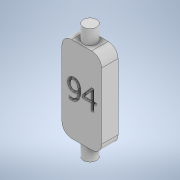
# Autodesk Inventor part: 16-2
Saved by Autodesk Inventor 2022 (Build 260153000, 153)
## iProperties
Created: 2021-09-25
Part Number: 16-2
Material: 일반
Document SubType Name: Modeling
Designer: 서울공업고등학교
Density: 1 g/cm^3
Appearance: 기본값
Author: 서울공업고등학교
Autodesk Inventor part; units mm, degrees
ref_plane "YZ Plane" through (0, 0, 0) normal (1, 0, 0) x (0, 1, 0)
ref_plane "XZ Plane" through (0, 0, 0) normal (0, 1, 0) x (-1, 0, 0)
ref_plane "XY Plane" through (0, 0, 0) normal (0, 0, 1) x (1, 0, 0)
sketch "스케치1" plane through (0, 0, 0) normal (0, 0, 1) x (1, 0, 0)
  line L0 (-6, 13) -> (6, 13)
  line L1 (6, 13) -> (6, -13)
  line L2 (6, -13) -> (-6, -13)
  line L3 (-6, -13) -> (-6, 13)
  line L4 (-6, 13) -> (6, -13) construction
  line L5 (6, 13) -> (-6, -13) construction
  point P0 (0, 0)
  dimension "d0" = 12
  dimension "d1" = 26
  constraints: 12 end point, 2 midpoint, 2 parallel, 1 horizontal, 1 perpendicular
  measures "d0" distance of L1.end L2.end
  measures "d1" distance of L0.end L1.end
extrude "돌출1" add sketch "스케치1" along normal mid plane 5
fillet "모깎기1" radius 3 4 edges at (6, 13, 0) (-6, 13, 0) (6, -13, 0) (-6, -13, 0)
sketch "스케치2" plane through (-3, 13, 2.5) normal (0, 1, 0) x (1, 0, 0)
  circle A0 centre (3, 2.5) radius 2
  dimension "d5" = 4
  constraints: 1 centre point, 1 coincident
  measures "d5" diameter of A0
extrude "돌출2" add sketch "스케치2" along normal blind 4.5 and the other way blind 30.5
sketch "스케치3" plane through (0, 0, 2.5) normal (0, 0, 1) x (1, 0, 0)
  line L0 (-4.5251, 3.4564) -> (4.6298, 3.4564) construction
  line L1 (4.6298, 3.4564) -> (4.6298, -2.8858) construction
  line L2 (4.6298, -2.8858) -> (-4.5251, -2.8858) construction
  line L3 (-4.5251, -2.8858) -> (-4.5251, 3.4564) construction
  spline S0 degree 2 poles (-4.2483, 1.3506) (-4.2483, 1.8202) (-3.9418, 2.6012) (-3.6749, 2.883) knots 0 0 0 1 2 2 2
  spline S1 degree 2 poles (-3.6749, 2.883) (-3.4228, 3.1549) (-2.6863, 3.4564) (-2.3106, 3.4564) knots 0 0 0 1 2 2 2
  spline S2 degree 2 poles (-2.3106, 3.4564) (-1.8904, 3.4564) (-1.2082, 3.1746) (-0.9561, 2.9077) knots 0 0 0 1 2 2 2
  spline S3 degree 2 poles (-0.9561, 2.9077) (-0.6397, 2.5715) (-0.2937, 1.484) (-0.2937, 0.6486) knots 0 0 0 1 2 2 2
  spline S4 degree 2 poles (-0.2937, 0.6486) (-0.2937, -0.1077) (-0.6348, -1.4622) (-0.966, -1.912) knots 0 0 0 1 2 2 2
  spline S5 degree 2 poles (-0.966, -1.912) (-1.317, -2.3866) (-2.3056, -2.8858) (-3.0273, -2.8858) knots 0 0 0 1 2 2 2
  spline S6 degree 2 poles (-3.0273, -2.8858) (-3.1905, -2.8858) (-3.5612, -2.8512) (-3.7194, -2.8018) knots 0 0 0 1 2 2 2
  line L4 (-3.7194, -2.8018) -> (-3.7194, -2.0158)
  line L5 (-3.7194, -2.0158) -> (-3.6798, -2.0158)
  spline S7 degree 2 poles (-3.6798, -2.0158) (-3.576, -2.0751) (-3.141, -2.1789) (-2.9186, -2.1789) knots 0 0 0 1 2 2 2
  spline S8 degree 2 poles (-2.9186, -2.1789) (-2.1178, -2.1789) (-1.2033, -1.1211) (-1.139, -0.1423) knots 0 0 0 1 2 2 2
  spline S9 degree 2 poles (-1.139, -0.1423) (-1.4653, -0.3648) (-2.0585, -0.5674) (-2.4094, -0.5674) knots 0 0 0 1 2 2 2
  spline S10 degree 2 poles (-2.4094, -0.5674) (-2.7456, -0.5674) (-3.3042, -0.4191) (-3.5859, -0.2066) knots 0 0 0 1 2 2 2
  spline S11 degree 2 poles (-3.5859, -0.2066) (-3.9122, 0.0455) (-4.2483, 0.8117) (-4.2483, 1.3506) knots 0 0 0 1 2 2 2
  spline S12 degree 2 poles (-1.1192, 0.8315) (-1.1192, 1.4494) (-1.3466, 2.2305) (-1.5493, 2.443) knots 0 0 0 1 2 2 2
  spline S13 degree 2 poles (-1.5493, 2.443) (-1.7273, 2.6408) (-2.098, 2.7891) (-2.3155, 2.7891) knots 0 0 0 1 2 2 2
  spline S14 degree 2 poles (-2.3155, 2.7891) (-2.8197, 2.7891) (-3.4179, 2.0673) (-3.4179, 1.3852) knots 0 0 0 1 2 2 2
  spline S15 degree 2 poles (-3.4179, 1.3852) (-3.4179, 0.9996) (-3.2201, 0.5003) (-3.0026, 0.3224) knots 0 0 0 1 2 2 2
  spline S16 degree 2 poles (-3.0026, 0.3224) (-2.8444, 0.1938) (-2.4539, 0.1098) (-2.2265, 0.1098) knots 0 0 0 1 2 2 2
  spline S17 degree 2 poles (-2.2265, 0.1098) (-1.9645, 0.1098) (-1.3615, 0.2927) (-1.1341, 0.4459) knots 0 0 0 1 2 2 2
  spline S18 degree 2 poles (-1.1341, 0.4459) (-1.1291, 0.5053) (-1.1192, 0.7079) (-1.1192, 0.8315) knots 0 0 0 1 2 2 2
  line L6 (4.4222, -0.6712) -> (3.6955, -0.6712)
  line L7 (3.6955, -0.6712) -> (3.6955, -2.7672)
  line L8 (3.6955, -2.7672) -> (2.9095, -2.7672)
  line L9 (2.9095, -2.7672) -> (2.9095, -0.6712)
  line L10 (2.9095, -0.6712) -> (0.2155, -0.6712)
  line L11 (0.2155, -0.6712) -> (0.2155, 0.1889)
  line L12 (0.2155, 0.1889) -> (2.9441, 3.3328)
  line L13 (2.9441, 3.3328) -> (3.6955, 3.3328)
  line L14 (3.6955, 3.3328) -> (3.6955, -0.0138)
  line L15 (3.6955, -0.0138) -> (4.4222, -0.0138)
  line L16 (4.4222, -0.0138) -> (4.4222, -0.6712)
  line L17 (2.9095, -0.0138) -> (2.9095, 2.3689)
  line L18 (2.9095, 2.3689) -> (0.8581, -0.0138)
  line L19 (0.8581, -0.0138) -> (2.9095, -0.0138)
  point P0 (0, 0)
  constraints: 2 other
extrude "돌출3" cut sketch "스케치3" against normal blind 1
